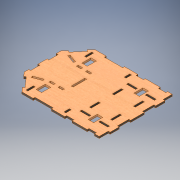
# Autodesk Inventor part: topCase
Saved by Autodesk Inventor 2019 (Build 230136000, 136)
## iProperties
Created: 2021-01-03
Part Number: topCase
Material: Дерево (вишня)
Document SubType Name: Modeling
Designer: Professional
Density: 0.63 g/cm^3
Appearance: Вишневое дерево — натуральный — со слабым глянцем
Author: Professional
Autodesk Inventor part; units mm, degrees
ref_plane "YZ Plane" through (0, 0, 0) normal (1, 0, 0) x (0, 1, 0)
ref_plane "XZ Plane" through (0, 0, 0) normal (0, 1, 0) x (-1, 0, 0)
ref_plane "XY Plane" through (0, 0, 0) normal (0, 0, 1) x (1, 0, 0)
sketch "Эскиз1" plane through (0, 0, 0) normal (0, 1, 0) x (-1, 0, 0)
  line L0 (-104, 0) -> (-104, -15)
  line L1 (-104, -15) -> (-100, -15)
  line L2 (-100, -15) -> (-100, -40)
  line L3 (-100, -40) -> (-104, -40)
  line L4 (-104, -40) -> (-104, -60)
  line L5 (-104, -60) -> (-100, -60)
  line L6 (-100, -60) -> (-100, -80)
  line L7 (-100, -80) -> (-90, -80)
  line L8 (-90, -80) -> (-90, -76)
  line L9 (-90, -76) -> (-74, -76)
  line L10 (-74, -76) -> (-74, -80)
  line L11 (-74, -80) -> (-41, -80)
  line L12 (-41, -80) -> (-41, -76)
  line L13 (-41, -76) -> (-25, -76)
  line L14 (-25, -76) -> (-25, -80)
  line L15 (-25, -80) -> (4.5, -80)
  line L16 (4.5, -80) -> (4.5, -76)
  line L17 (4.5, -76) -> (44.5, -76)
  line L18 (44.5, -76) -> (44.5, -80)
  line L19 (44.5, -80) -> (69, -80)
  line L20 (69, -80) -> (77, -70.8571)
  line L21 (77, -70.8571) -> (73.9897, -68.2231)
  line L22 (73.9897, -68.2231) -> (92.9897, -46.5088)
  line L23 (92.9897, -46.5088) -> (96, -49.1429)
  line L24 (96, -49.1429) -> (104, -40)
  line L25 (104, -40) -> (104, -30)
  line L26 (104, -30) -> (100, -30)
  line L27 (100, -30) -> (100, -10)
  line L28 (100, -10) -> (104, -10)
  line L29 (104, -10) -> (104, 0)
  line L30 (104, 0) -> (-104, 0)
  line L31 (68, -72) -> (64, -72)
  line L32 (64, -72) -> (64, -56)
  line L33 (64, -56) -> (68, -56)
  line L34 (68, -56) -> (68, -72)
  line L35 (-15, -72) -> (-19, -72)
  line L36 (-19, -72) -> (-19, -60)
  line L37 (-19, -60) -> (-15, -60)
  line L38 (-15, -60) -> (-15, -72)
  line L39 (-31, -49) -> (-51, -49)
  line L40 (-51, -49) -> (-51, -53)
  line L41 (-51, -53) -> (-31, -53)
  line L42 (-31, -53) -> (-31, -49)
  line L43 (-72, -53) -> (-92, -53)
  line L44 (-92, -53) -> (-92, -49)
  line L45 (-92, -49) -> (-72, -49)
  line L46 (-72, -49) -> (-72, -53)
  line L47 (-33.8, -35) -> (-37.8, -35)
  line L48 (-37.8, -35) -> (-37.8, -15)
  line L49 (-37.8, -15) -> (-33.8, -15)
  line L50 (-33.8, -15) -> (-33.8, -35)
  line L51 (-80.2, -35) -> (-84.2, -35)
  line L52 (-84.2, -35) -> (-84.2, -15)
  line L53 (-84.2, -15) -> (-80.2, -15)
  line L54 (-80.2, -15) -> (-80.2, -35)
  line L55 (-104, 0) -> (-104, 15)
  line L56 (-104, 15) -> (-100, 15)
  line L57 (-100, 15) -> (-100, 40)
  line L58 (-100, 40) -> (-104, 40)
  line L59 (-104, 40) -> (-104, 60)
  line L60 (-104, 60) -> (-100, 60)
  line L61 (-100, 60) -> (-100, 80)
  line L62 (-100, 80) -> (-90, 80)
  line L63 (-90, 80) -> (-90, 76)
  line L64 (-90, 76) -> (-74, 76)
  line L65 (-74, 76) -> (-74, 80)
  line L66 (-74, 80) -> (-41, 80)
  line L67 (-41, 80) -> (-41, 76)
  line L68 (-41, 76) -> (-25, 76)
  line L69 (-25, 76) -> (-25, 80)
  line L70 (-25, 80) -> (4.5, 80)
  line L71 (4.5, 80) -> (4.5, 76)
  line L72 (4.5, 76) -> (44.5, 76)
  line L73 (44.5, 76) -> (44.5, 80)
  line L74 (44.5, 80) -> (69, 80)
  line L75 (69, 80) -> (77, 70.8571)
  line L76 (77, 70.8571) -> (73.9897, 68.2231)
  line L77 (73.9897, 68.2231) -> (92.9897, 46.5088)
  line L78 (92.9897, 46.5088) -> (96, 49.1429)
  line L79 (96, 49.1429) -> (104, 40)
  line L80 (104, 40) -> (104, 30)
  line L81 (104, 30) -> (100, 30)
  line L82 (100, 30) -> (100, 10)
  line L83 (100, 10) -> (104, 10)
  line L84 (104, 10) -> (104, 0)
  line L85 (68, 72) -> (64, 72)
  line L86 (64, 72) -> (64, 56)
  line L87 (64, 56) -> (68, 56)
  line L88 (68, 56) -> (68, 72)
  line L89 (-15, 72) -> (-19, 72)
  line L90 (-19, 72) -> (-19, 60)
  line L91 (-19, 60) -> (-15, 60)
  line L92 (-15, 60) -> (-15, 72)
  line L93 (-31, 49) -> (-51, 49)
  line L94 (-51, 49) -> (-51, 53)
  line L95 (-51, 53) -> (-31, 53)
  line L96 (-31, 53) -> (-31, 49)
  line L97 (-72, 53) -> (-92, 53)
  line L98 (-92, 53) -> (-92, 49)
  line L99 (-92, 49) -> (-72, 49)
  line L100 (-72, 49) -> (-72, 53)
  line L101 (-33.8, 35) -> (-37.8, 35)
  line L102 (-37.8, 35) -> (-37.8, 15)
  line L103 (-37.8, 15) -> (-33.8, 15)
  line L104 (-33.8, 15) -> (-33.8, 35)
  line L105 (-80.2, 35) -> (-84.2, 35)
  line L106 (-84.2, 35) -> (-84.2, 15)
  line L107 (-84.2, 15) -> (-80.2, 15)
  line L108 (-80.2, 15) -> (-80.2, 35)
  point P0 (0, 0)
  point P1 (0, 0)
  dimension "d0" = 25
  dimension "d1" = 20
  dimension "d2" = 20
  dimension "d3" = 15
  dimension "d4" = 10
  dimension "d5" = 16
  dimension "d6" = 16
  dimension "d7" = 33
  dimension "d8" = 29.5
  dimension "d9" = 40
  dimension "d10" = 24.5
  dimension "d11" = 20
  dimension "d12" = 10
  dimension "d13" = 40
  dimension "d14" = 35
  dimension "d15" = 4
  dimension "d16" = 8
  dimension "d17" = 8
  dimension "d18" = 1
  dimension "d19" = 16
  dimension "d20" = 8
  dimension "d21" = 8
  dimension "d22" = 12
  dimension "d23" = 6
  dimension "d24" = 20
  dimension "d25" = 21
  dimension "d26" = 12
  dimension "d27" = 27
  dimension "d28" = 14
  dimension "d29" = 20
  dimension "d30" = 2.8
  dimension "d31" = 42.4
  constraints: 218 end point, 53 symmetric about line, 26 perpendicular, 20 point on line, 13 parallel, 10 equal length, 9 horizontal, 5 horizontal alignment, 4 vertical, 2 vertical alignment, 1 coincident, 1 midpoint
  measures "d0" distance between parallel lines of L1 L3
  measures "d1" distance between parallel lines of L7 L5
  measures "d2" distance between parallel lines of L5 L3
  measures "d3" distance between parallel lines of L30 L1
  measures "d4" distance between parallel lines of L6 L8
  measures "d5" distance between parallel lines of L8 L10
  measures "d6" distance between parallel lines of L12 L14
  measures "d7" distance between parallel lines of L10 L12
  measures "d8" distance between parallel lines of L14 L16
  measures "d9" distance between parallel lines of L16 L18
  measures "d10" distance from line of L18 L19.end
  measures "d11" distance between parallel lines of L26 L28
  measures "d12" distance between parallel lines of L30 L28
  measures "d13" vertical distance of L24.end L19.end
  measures "d14" horizontal distance of L19.end L24.end
  measures "d15" distance of L27.end L28.end
  measures "d16" horizontal distance of L20.end L19.end
  measures "d17" horizontal distance of L24.end L23.end
  measures "d18" horizontal distance of L19.end L31.start
  measures "d19" distance between parallel lines of L33 L31
  measures "d20" distance between parallel lines of L19 L31
  measures "d21" distance between parallel lines of L15 L35
  measures "d22" distance between parallel lines of L37 L35
  measures "d23" horizontal distance of L35.end L14.end
  measures "d24" distance between parallel lines of L40 L42
  measures "d25" distance between parallel lines of L46 L40
  measures "d26" distance from line of L36.end L42
  measures "d27" distance between parallel lines of L11 L41
  measures "d28" distance between parallel lines of L39 L47
  measures "d29" distance between parallel lines of L49 L47
  measures "d30" distance between parallel lines of L50 L42
  measures "d31" distance between parallel lines of L54 L48
extrude "Выдавливание1" add sketch "Эскиз1" along normal blind 4
sketch "Эскиз2" plane through (0, 4, 0) normal (0, 1, 0) x (1, 0, 0)
  line L0 (-58, -32) -> (-48, -32)
  line L1 (-48, -32) -> (-48, -28)
  line L2 (-48, -28) -> (-58, -28)
  line L3 (-58, -28) -> (-58, -32)
  line L4 (-67.3144, -35.6469) -> (-86.1083, -42.4873)
  line L5 (-86.1083, -42.4873) -> (-87.4764, -38.7285)
  line L6 (-87.4764, -38.7285) -> (-68.6825, -31.8881)
  line L7 (-68.6825, -31.8881) -> (-67.3144, -35.6469)
  line L8 (-104, 10) -> (-104, -10) projected
  line L9 (-104, 0) -> (104, 0)
  line L10 (104, -15) -> (104, 15) projected
  line L11 (-58, 32) -> (-48, 32)
  line L12 (-48, 32) -> (-48, 28)
  line L13 (-48, 28) -> (-58, 28)
  line L14 (-58, 28) -> (-58, 32)
  line L15 (-67.3144, 35.6469) -> (-86.1083, 42.4873)
  line L16 (-86.1083, 42.4873) -> (-87.4764, 38.7285)
  line L17 (-87.4764, 38.7285) -> (-68.6825, 31.8881)
  line L18 (-68.6825, 31.8881) -> (-67.3144, 35.6469)
  line L19 (-38, -32) -> (-28, -32)
  line L20 (-28, -32) -> (-28, -28)
  line L21 (-28, -28) -> (-38, -28)
  line L22 (-38, -28) -> (-38, -32)
  line L23 (-38, 32) -> (-28, 32)
  line L24 (-28, 32) -> (-28, 28)
  line L25 (-28, 28) -> (-38, 28)
  line L26 (-38, 28) -> (-38, 32)
  line L27 (68, -60) -> (56, -60)
  line L28 (56, -60) -> (56, -40)
  line L29 (56, -40) -> (68, -40)
  line L30 (68, -40) -> (68, -60)
  line L31 (51, -49) -> (51, -53) projected
  line L32 (41, -80) -> (74, -80) projected
  line L33 (68, 60) -> (56, 60)
  line L34 (56, 60) -> (56, 40)
  line L35 (56, 40) -> (68, 40)
  line L36 (68, 40) -> (68, 60)
  line L37 (-46, -60) -> (-58, -60)
  line L38 (-58, -60) -> (-58, -40)
  line L39 (-58, -40) -> (-46, -40)
  line L40 (-46, -40) -> (-46, -60)
  line L41 (-64, -56) -> (-64, -72) projected
  line L42 (-46, 60) -> (-58, 60)
  line L43 (-58, 60) -> (-58, 40)
  line L44 (-58, 40) -> (-46, 40)
  line L45 (-46, 40) -> (-46, 60)
  line L46 (-26, -15) -> (-22, -15)
  line L47 (-22, -15) -> (-22, 15)
  line L48 (-22, 15) -> (-26, 15)
  line L49 (-26, 15) -> (-26, -15)
  point P0 (0, 0)
  dimension "d34" = 20
  dimension "d35" = 56
  dimension "d36" = 4
  dimension "d39" = 10
  dimension "d40" = 20
  dimension "d42" = 10
  dimension "d48" = 10
  dimension "d49" = 10
  dimension "d51" = 12
  dimension "d52" = 20
  dimension "d53" = 5
  dimension "d54" = 20
  dimension "d55" = 12
  dimension "d56" = 6
  dimension "d57" = 30
  dimension "d58" = 2
  constraints: 90 end point, 21 symmetric about line, 12 parallel, 6 perpendicular, 5 horizontal, 4 equal length, 2 coincident, 2 horizontal alignment, 2 midpoint, 2 point on line, 1 vertical alignment, 1 other
  measures "d34" angle of L9 L6
  measures "d35" diameter of L2 L9
  measures "d36" distance between parallel lines of L4 L6
  measures "d39" distance between parallel lines of L1 L3
  measures "d40" distance between parallel lines of L5 L7
  measures "d42" distance from line of L7 L0.start
  measures "d48" distance between parallel lines of L20 L22
  measures "d49" distance between parallel lines of L1 L22
  measures "d51" distance between parallel lines of L28 L30
  measures "d52" distance between parallel lines of L27 L29
  measures "d53" distance between parallel lines of L31 L28
  measures "d54" distance between parallel lines of L32 L27
  measures "d55" distance between parallel lines of L38 L40
  measures "d56" distance between parallel lines of L41 L38
  measures "d57" distance between parallel lines of L46 L48
  measures "d58" distance from line of L23.end L49
extrude "Выдавливание2" cut sketch "Эскиз2" against normal through all
